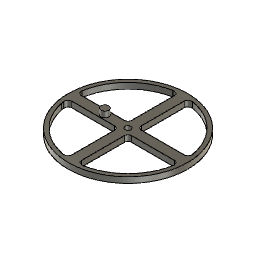
spinning_part_62mm_diameter v2 (Autodesk Fusion 360 design; units mm, degrees)
Autodesk Fusion 360 part; units mm, degrees
sketch "Sketch1" plane through (0, 0, 0) normal (0, 0, 1) x (1, 0, 0)
  circle A0 centre (0, 0) radius 31
  line L0 (-2.5, 4.5) -> (-2.5, 26.6021)
  line L1 (2.5, 26.6069) -> (2.5, 4.5)
  line L2 (4.5, 2.5) -> (26.6004, 2.5)
  line L3 (30, 2.5) -> (30, -2.5)
  line L4 (26.6004, -2.5) -> (4.5, -2.5)
  line L5 (-2.5, -4.5) -> (-2.5, -26.5963)
  line L6 (-2.5, -29.8321) -> (2.5, -29.8321)
  line L7 (2.5, -26.5963) -> (2.5, -4.5)
  line L8 (-4.5, -2.5) -> (-26.5729, -2.5)
  line L9 (-30.0038, -2.5) -> (-30.0038, 2.5)
  line L10 (-26.6252, 2.5) -> (-4.5, 2.5)
  arc A1 (2.5, 4.5) -> (4.5, 2.5) centre (4.5, 4.5) ccw
  arc A2 (4.5, -2.5) -> (2.5, -4.5) centre (4.5, -4.5) ccw
  arc A3 (-2.5, -4.5) -> (-4.5, -2.5) centre (-4.5, -4.5) ccw
  arc A4 (-4.5, 2.5) -> (-2.5, 4.5) centre (-4.5, 4.5) ccw
  line L11 (-28.6096, 4.7492) -> (-28.6133, 4.7201)
  arc A5 (-28.6096, 4.7492) -> (-26.6252, 2.5) centre (-26.6252, 4.5) ccw
  line L12 (-28.5511, -4.794) -> (-28.3705, -6.0097)
  arc A6 (-26.5729, -2.5) -> (-28.5511, -4.794) centre (-26.5729, -4.5) ccw
  line L13 (-4.7741, -28.5774) -> (-5.4383, -28.4855)
  line L14 (4.7741, -28.5774) -> (5.4383, -28.4855)
  arc A7 (2.5, -26.5963) -> (4.7741, -28.5774) centre (4.5, -26.5963) ccw
  arc A8 (-4.7741, -28.5774) -> (-2.5, -26.5963) centre (-4.5, -26.5963) ccw
  line L15 (28.582, -4.7706) -> (28.5047, -5.3371)
  line L16 (28.582, 4.7706) -> (28.5047, 5.3371)
  arc A9 (26.6004, 2.5) -> (28.582, 4.7706) centre (26.6004, 4.5) ccw
  arc A10 (28.582, -4.7706) -> (26.6004, -2.5) centre (26.6004, -4.5) ccw
  line L17 (4.765, 28.5892) -> (5.177, 28.5342)
  arc A11 (4.765, 28.5892) -> (2.5, 26.6069) centre (4.5, 26.6069) ccw
  line L18 (-4.7691, 28.5839) -> (-5.2948, 28.5125)
  arc A12 (-2.5, 26.6021) -> (-4.7691, 28.5839) centre (-4.5, 26.6021) ccw
  arc A13 (28.5047, 5.3371) -> (5.177, 28.5342) centre (0, 0) ccw
  arc A14 (-5.2948, 28.5125) -> (-28.6133, 4.7201) centre (0, 0) ccw
  arc A15 (-28.3705, -6.0097) -> (-5.4383, -28.4855) centre (0, 0) ccw
  arc A16 (5.4383, -28.4855) -> (28.5047, -5.3371) centre (0, 0) ccw
  circle A17 centre (0, 0) radius 1.5
  dimension "d1" = 62
  dimension "d2" = 58
  dimension "d7" = 2
  dimension "d8" = 2
  dimension "d9" = 2
  dimension "d10" = 2
  dimension "d11" = 2
  dimension "d12" = 2
  dimension "d13" = 2
  dimension "d14" = 2
  dimension "d15" = 2
  dimension "d16" = 2
  dimension "d17" = 2
  dimension "d18" = 2
  dimension "d19" = 3
  constraint concentric A0 A13
  constraint vertical L0
  constraint vertical L1
  constraint horizontal L2
  constraint vertical L3
  constraint horizontal L4
  constraint vertical L5
  constraint horizontal L6
  constraint vertical L7
  constraint horizontal L8
  constraint vertical L9
  constraint horizontal L10
  constraint tangent L1 A1
  constraint tangent L2 A1
  constraint tangent L7 A2
  constraint tangent L4 A2
  constraint tangent L8 A3
  constraint tangent L5 A3
  constraint tangent L0 A4
  constraint tangent L10 A4
  constraint coincident L11.end A13
  constraint coincident L9.end L10
  constraint tangent L11 A5
  constraint tangent L10 A5
  constraint coincident L12.end A13
  constraint coincident L9.start L8
  constraint tangent L12 A6
  constraint tangent L8 A6
  constraint coincident L13.end A13
  constraint coincident L14.end A13
  constraint coincident L6.end L7
  constraint tangent L14 A7
  constraint tangent L7 A7
  constraint coincident L6.start L5
  constraint tangent L13 A8
  constraint tangent L5 A8
  constraint coincident L3.start L2
  constraint tangent L16 A9
  constraint tangent L2 A9
  constraint coincident L3.end L4
  constraint tangent L15 A10
  constraint tangent L4 A10
  constraint tangent L1 A11
  constraint tangent L17 A11
  constraint coincident L18.end A13
  constraint tangent L18 A12
  constraint tangent L0 A12
  constraint concentric A13 A14
  constraint concentric A14 A15
  constraint concentric A15 A16
  constraint concentric A0 A17
  measures "d1" diameter of A0
  measures "d2" diameter of A13
  measures "d7" radius of A1
  measures "d8" radius of A2
  measures "d9" radius of A3
  measures "d10" radius of A4
  measures "d11" radius of A5
  measures "d12" radius of A6
  measures "d13" radius of A7
  measures "d14" radius of A8
  measures "d15" radius of A9
  measures "d16" radius of A10
  measures "d17" radius of A11
  measures "d18" radius of A12
  measures "d19" diameter of A17
extrude "Extrude1" add sketch "Sketch1" along normal blind 3 makes body 1
sketch "Sketch2" plane through (0, 0, 3) normal (0, 0, 1) x (-1, 0, 0)
  line L0 (4.5, -2.5) -> (26.6252, -2.5)
  arc A0 (28.6126, -4.7241) -> (26.6252, -2.5) centre (26.6252, -4.5) ccw
  arc A1 (28.6126, -4.7241) -> (28.6133, -4.7201) centre (0, 0) ccw
  line L1 (28.6133, -4.7201) -> (28.6096, -4.7492)
  arc A2 (28.6096, -4.7492) -> (28.6126, -4.7241) centre (26.6252, -4.5) ccw
  arc A3 (5.2948, -28.5125) -> (28.6126, -4.7241) centre (0, 0) ccw
  line L2 (5.2948, -28.5125) -> (4.7691, -28.5839)
  arc A4 (2.5, -26.6021) -> (4.7691, -28.5839) centre (4.5, -26.6021) ccw
  line L3 (2.5, -26.6021) -> (2.5, -4.5)
  arc A5 (4.5, -2.5) -> (2.5, -4.5) centre (4.5, -4.5) ccw
  arc A6 (2.5, 4.5) -> (4.5, 2.5) centre (4.5, 4.5) ccw
  line L4 (2.5, 4.5) -> (2.5, 26.5963)
  arc A7 (4.7741, 28.5774) -> (2.5, 26.5963) centre (4.5, 26.5963) ccw
  line L5 (4.7741, 28.5774) -> (5.4383, 28.4855)
  arc A8 (28.3705, 6.0097) -> (5.4383, 28.4855) centre (0, 0) ccw
  line L6 (28.3705, 6.0097) -> (28.5511, 4.794)
  arc A9 (26.5729, 2.5) -> (28.5511, 4.794) centre (26.5729, 4.5) ccw
  line L7 (26.5729, 2.5) -> (4.5, 2.5)
  circle A10 centre (0, 0) radius 1.5
  arc A11 (-4.765, -28.5892) -> (-2.5, -26.6069) centre (-4.5, -26.6069) ccw
  line L8 (-4.765, -28.5892) -> (-5.177, -28.5342)
  arc A12 (-28.5047, -5.3371) -> (-5.177, -28.5342) centre (0, 0) ccw
  line L9 (-28.5047, -5.3371) -> (-28.582, -4.7706)
  arc A13 (-26.6004, -2.5) -> (-28.582, -4.7706) centre (-26.6004, -4.5) ccw
  line L10 (-26.6004, -2.5) -> (-4.5, -2.5)
  arc A14 (-2.5, -4.5) -> (-4.5, -2.5) centre (-4.5, -4.5) ccw
  line L11 (-2.5, -4.5) -> (-2.5, -26.6069)
  arc A15 (-2.5, 26.5963) -> (-4.7741, 28.5774) centre (-4.5, 26.5963) ccw
  line L12 (-2.5, 26.5963) -> (-2.5, 4.5)
  arc A16 (-4.5, 2.5) -> (-2.5, 4.5) centre (-4.5, 4.5) ccw
  line L13 (-4.5, 2.5) -> (-26.6004, 2.5)
  arc A17 (-28.582, 4.7706) -> (-26.6004, 2.5) centre (-26.6004, 4.5) ccw
  line L14 (-28.582, 4.7706) -> (-28.5047, 5.3371)
  arc A18 (-5.4383, 28.4855) -> (-28.5047, 5.3371) centre (0, 0) ccw
  line L15 (-5.4383, 28.4855) -> (-4.7741, 28.5774)
  circle A19 centre (0, 0) radius 31
  line L16 (31, 0) -> (12, 0)
  circle A20 centre (12, 0) radius 2
  dimension "d22" = 19
  dimension "d23" = 4
  constraint coincident A19 L16.start
  constraint coincident L16.end A20.centre
  measures "d22" distance of L16.start L16.end
  measures "d23" diameter of A20
extrude "Extrude2" add sketch "Sketch2" along normal blind 3 separate body contours A20 makes body 2
